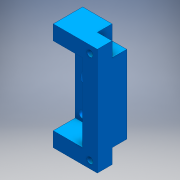
# Autodesk Inventor part: powerSwitchHolder
Saved by Autodesk Inventor 2016 (Build 200138000, 138)
## iProperties
Created: 2016-06-13
Part Number: powerSwitchHolder
Material: Generic
Document SubType Name: Modeling
Designer: hesaon
Density: 1 g/cm^3
Appearance: Default
Author: hesaon
Autodesk Inventor part; units mm, degrees
ref_plane "YZ Plane" through (0, 0, 0) normal (1, 0, 0) x (0, 1, 0)
ref_plane "XZ Plane" through (0, 0, 0) normal (0, 1, 0) x (-1, 0, 0)
ref_plane "XY Plane" through (0, 0, 0) normal (0, 0, 1) x (1, 0, 0)
sketch "Sketch1" plane through (0, 0, 0) normal (0, 1, 0) x (-1, 0, 0)
  line L0 (0, 0) -> (20, 0)
  line L1 (20, 0) -> (20, -73)
  line L2 (20, -73) -> (0, -73)
  line L3 (0, -73) -> (0, 0)
  circle A0 centre (10, -36.5) radius 6.25
  dimension "d0" = 20
  dimension "d1" = 73
  dimension "d2" = 12.5
  dimension "d3" = 10
  dimension "d4" = 36.5
  constraints: 8 end point, 2 parallel, 1 centre point, 1 horizontal, 1 perpendicular
  measures "d0" distance of L1.end L2.end
  measures "d1" distance of L0.end L1.end
  measures "d2" diameter of A0
  measures "d3" distance from line of L3 A0.centre
  measures "d4" distance from line of L2 A0.centre
extrude "Extrusion1" add sketch "Sketch1" along normal blind 5
sketch "Sketch2" plane through (0, 0, 0) normal (1, 0, 0) x (0, 0, -1)
  line L0 (10, 5) -> (63, 5)
  line L1 (63, 5) -> (63, -15)
  line L2 (63, -15) -> (10, -15)
  line L3 (10, -15) -> (10, 5)
  line L4 (0, 5) -> (73, 5) projected
  line L5 (0, 0) -> (0, 5) projected
  line L6 (73, 0) -> (73, 5) projected
  line L7 (73, 0) -> (0, 0) projected
  dimension "d7" = 10
  dimension "d8" = 10
  dimension "d9" = 15
  constraints: 8 end point, 2 parallel, 1 collinear, 1 horizontal, 1 perpendicular
  measures "d7" distance between parallel lines of L5 L3
  measures "d8" distance between parallel lines of L6 L1
  measures "d9" distance between parallel lines of L7 L2
extrude "Extrusion2" add sketch "Sketch2" along normal blind 10 contours L0 L1 L7 L3 | L7 L1 L2 L3
sketch "Sketch3" plane through (0, -15, -10) normal (0, 0, 1) x (1, 0, 0)
  line L0 (0, 10) -> (10, 10)
  line L1 (10, 10) -> (10, 0)
  line L2 (10, 0) -> (0, 0)
  line L3 (0, 0) -> (0, 10)
  line L4 (10, 20) -> (10, 0) projected
  line L5 (0, 0) -> (10, 0) projected
  point P0 (0, 15)
  dimension "d12" = 10
  dimension "d13" = 10
  constraints: 8 end point, 2 collinear, 2 parallel, 1 horizontal, 1 perpendicular
  measures "d12" distance of L1.end L2.end
  measures "d13" distance of L0.end L1.end
extrude "Extrusion3" add sketch "Sketch3" along normal blind 10
sketch "Sketch4" plane through (0, 0, 0) normal (0, -1, 0) x (1, 0, 0)
  line L0 (-20, -10) -> (0, -10)
  line L1 (0, -10) -> (0, 0)
  line L2 (0, 0) -> (-20, 0)
  line L3 (-20, 0) -> (-20, -10)
  line L4 (0, 0) -> (-20, 0) projected
  line L5 (-20, 0) -> (-20, -73) projected
  line L6 (0, -63) -> (0, 0) projected
  dimension "d16" = 10
  constraints: 8 end point, 3 collinear, 2 parallel, 1 horizontal, 1 perpendicular
  measures "d16" distance between parallel lines of L2 L0
extrude "Extrusion4" add sketch "Sketch4" along normal blind 15
sketch "Sketch5" plane through (0, -15, -63) normal (0, 0, -1) x (-1, 0, 0)
  line L0 (-10, 0) -> (-10, 10) projected
  line L1 (-10, 0) -> (-10, 10)
  line L2 (0, 10) -> (-10, 10) projected
  line L3 (-10, 10) -> (0, 10)
  line L4 (0, 10) -> (0, 15)
  line L5 (0, 10) -> (0, 20) projected
  line L6 (0, 15) -> (20, 15) projected
  line L7 (-10, 0) -> (20, 0) projected
  line L8 (20, 15) -> (20, 0)
  line L9 (20, 0) -> (-10, 0)
  dimension "d19" = 15
  constraints: 10 end point, 2 collinear, 2 vertical, 1 perpendicular
  measures "d19" distance between parallel lines of L7 L6
extrude "Extrusion5" add sketch "Sketch5" along normal blind 10
sketch "Sketch6" plane through (0, 5, 0) normal (0, 1, 0) x (1, 0, 0)
  line L0 (-5, 58.5) -> (-15, 58.5) construction
  line L1 (-5, 61) -> (-15, 61)
  line L2 (-15, 56) -> (-5, 56)
  arc A0 (-5, 56) -> (-5, 61) centre (-5, 58.5) ccw
  arc A1 (-15, 61) -> (-15, 56) centre (-15, 58.5) ccw
  line L3 (-5, 14.5) -> (-15, 14.5) construction
  line L4 (-5, 17) -> (-15, 17)
  line L5 (-15, 12) -> (-5, 12)
  arc A2 (-5, 12) -> (-5, 17) centre (-5, 14.5) ccw
  arc A3 (-15, 17) -> (-15, 12) centre (-15, 14.5) ccw
  line L6 (-20, 0) -> (0, 0) projected
  line L7 (0, 73) -> (-20, 73) projected
  line L8 (-20, 73) -> (-20, 0) projected
  point P0 (-10, 58.5)
  point P1 (-10, 14.5)
  dimension "d22" = 5
  dimension "d23" = 5
  dimension "d24" = 12
  dimension "d25" = 12
  dimension "d26" = 10
  dimension "d27" = 10
  dimension "d28" = 10
  dimension "d29" = 10
  constraints: 16 end point, 8 point on circle, 8 tangent, 4 centre point, 3 parallel, 2 midpoint, 1 horizontal
  measures "d22" distance between parallel lines of L4 L5
  measures "d23" distance between parallel lines of L1 L2
  measures "d24" distance between parallel lines of L6 L5
  measures "d25" distance between parallel lines of L7 L1
  measures "d26" distance from line of L8 point (-10, 58.5)
  measures "d27" distance from line of L8 point (-10, 14.5)
  measures "d28" distance of L3.end L3.start
  measures "d29" distance of L0.end L0.start
extrude "Extrusion6" cut sketch "Sketch6" against normal blind 10
hole "Hole1" at (5, -5, -5) direction (0, -1, 0) diameter 4.2 end through all
hole "Hole3" at (5, -5, -68) direction (0, -1, 0) diameter 4.2 end through all
body "Solid1"
